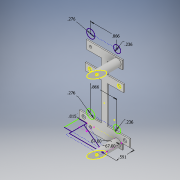
# Autodesk Inventor part: PI Rfid baracke angled reconfig
Saved by Autodesk Inventor 2018 (Build 220112000, 112)
## iProperties
Created: 2019-09-27
Part Number: PI Rfid baracke angled reconfig
Material: Generic
Document SubType Name: Modeling
Designer: Jacob
Density: 1 g/cm^3
Appearance: Default
Author: Jacob
Autodesk Inventor part; units mm, degrees
ref_plane "YZ Plane" through (0, 0, 0) normal (1, 0, 0) x (0, 1, 0)
ref_plane "XZ Plane" through (0, 0, 0) normal (0, 1, 0) x (-1, 0, 0)
ref_plane "XY Plane" through (0, 0, 0) normal (0, 0, 1) x (1, 0, 0)
sketch "Sketch1" plane through (0, 0, 0) normal (0, 0, 1) x (1, 0, 0)
  line L0 (-2.5, 15.5) -> (2.5, 15.5)
  line L1 (2.5, 15.5) -> (2.5, -15.5)
  line L2 (2.5, -15.5) -> (-2.5, -15.5)
  line L3 (-2.5, -15.5) -> (-2.5, 15.5)
  line L4 (-2.5, 15.5) -> (2.5, -15.5) construction
  line L5 (2.5, 15.5) -> (-2.5, -15.5) construction
  line L6 (0, 0) -> (0, 29.5852) construction
  line L7 (-16, 21.5) -> (16, 21.5)
  line L8 (16, 21.5) -> (16, 15.5)
  line L9 (16, 15.5) -> (-16, 15.5)
  line L10 (-16, 15.5) -> (-16, 21.5)
  line L11 (-16, 21.5) -> (16, 15.5) construction
  line L12 (16, 21.5) -> (-16, 15.5) construction
  line L13 (0, 0) -> (0, -27.9929) construction
  line L14 (-21, -15.5) -> (21, -15.5)
  line L15 (21, -15.5) -> (21, -21.5)
  line L16 (21, -21.5) -> (-21, -21.5)
  line L17 (-21, -21.5) -> (-21, -15.5)
  line L18 (-21, -15.5) -> (21, -21.5) construction
  line L19 (21, -15.5) -> (-21, -21.5) construction
  line L20 (16, 18.5) -> (-16, 18.5) construction
  line L21 (21, -18.5) -> (-21, -18.5) construction
  point P0 (0, 18.5)
  point P1 (0, -18.5)
  dimension "d0" = 5
  dimension "d2" = 32
  dimension "d3" = 6
  dimension "d4" = 0
  dimension "d5" = 42
  dimension "d6" = 6
  dimension "d7" = 0
  dimension "d65" = 37
  constraints: 44 end point, 10 midpoint, 7 parallel, 3 horizontal, 3 perpendicular, 2 point on line, 1 vertical
  measures "d0" distance between parallel lines of L1 L3
  measures "d2" distance of L7.start L7.end
  measures "d3" distance of L7.end L8.end
  measures "d4" distance between parallel lines of L0 L9
  measures "d5" distance of L15.end L16.end
  measures "d6" distance of L14.end L15.end
  measures "d7" distance between parallel lines of L2 L14
  measures "d65" vertical distance of L21.start L20.start
extrude "Extrusion1" add sketch "Sketch1" along normal blind 1
sketch "Sketch2" plane through (0, 0, 1) normal (0, 0, 1) x (1, 0, 0)
  line L0 (-16, 21.5) -> (-16, 15.5) projected
  line L1 (-16, 18.5) -> (16, 18.5) construction
  line L2 (16, 15.5) -> (16, 21.5) projected
  line L3 (-21, -15.5) -> (-21, -21.5) projected
  line L4 (-21, -18.5) -> (21, -18.5) construction
  line L5 (21, -15.5) -> (21, -21.5) projected
  circle A0 centre (-17.25, -18.5) radius 1.5
  circle A1 centre (17.25, -18.5) radius 1.5
  line L6 (0, 0) -> (0, -21.5) construction
  line L7 (21, -21.5) -> (-21, -21.5) projected
  line L8 (0, 0) -> (0, 21.5) construction
  line L9 (16, 21.5) -> (-16, 21.5) projected
  circle A2 centre (-12.25, 18.5) radius 1.5
  circle A3 centre (12.25, 18.5) radius 1.5
  dimension "d10" = 34.5
  dimension "d13" = 17.25
  dimension "d14" = 17.25
  dimension "d15" = 3
  dimension "d16" = 3
  dimension "d17" = 24.5
  dimension "d18" = 12.25
  dimension "d19" = 12.25
  dimension "d20" = 3
  dimension "d21" = 3
  dimension "d66" = 37
  constraints: 8 end point, 6 midpoint, 4 centre point, 4 point on line
  measures "d10" distance of A1.centre A0.centre
  measures "d13" distance from line of L6 A0.centre
  measures "d14" distance from line of L6 A1.centre
  measures "d15" diameter of A0
  measures "d16" diameter of A1
  measures "d17" distance of A3.centre A2.centre
  measures "d18" distance from line of L8 A2.centre
  measures "d19" distance from line of L8 A3.centre
  measures "d20" diameter of A2
  measures "d21" diameter of A3
  measures "d66" distance between parallel lines of L4 L1
extrude "Extrusion2" cut sketch "Sketch2" against normal blind 2
sketch "Sketch4" plane through (0, 0, 1) normal (0, 0, 1) x (1, 0, 0)
  line L0 (0, 0) -> (0, 68.1033) construction
  line L1 (0, 0) -> (0, -40.1743) construction
  line L2 (-15, 38.5) -> (15, 38.5)
  line L3 (15, 38.5) -> (15, 31.5)
  line L4 (15, 31.5) -> (-15, 31.5)
  line L5 (-15, 31.5) -> (-15, 38.5)
  line L6 (-15, 38.5) -> (15, 31.5) construction
  line L7 (15, 38.5) -> (-15, 31.5) construction
  line L8 (-15, -19.5) -> (15, -19.5)
  line L9 (15, -19.5) -> (15, -26.5)
  line L10 (15, -26.5) -> (-15, -26.5)
  line L11 (-15, -26.5) -> (-15, -19.5)
  line L12 (-15, -19.5) -> (15, -26.5) construction
  line L13 (15, -19.5) -> (-15, -26.5) construction
  circle A0 centre (-17.25, -18.5) radius 1.5 projected
  line L14 (-2.5, 31.5) -> (2.5, 31.5)
  line L15 (2.5, 31.5) -> (2.5, 21.5)
  line L16 (2.5, 21.5) -> (-2.5, 21.5)
  line L17 (-2.5, 21.5) -> (-2.5, 31.5)
  line L18 (-2.5, 31.5) -> (2.5, 21.5) construction
  line L19 (2.5, 31.5) -> (-2.5, 21.5) construction
  line L20 (16, 21.5) -> (-16, 21.5) projected
  line L21 (-15, -23) -> (15, -23) construction
  line L22 (-15, 35) -> (15, 35) construction
  circle A1 centre (-11.5, -23) radius 1
  circle A2 centre (11.5, -23) radius 1
  circle A3 centre (-11.5, 35) radius 1
  circle A4 centre (11.5, 35) radius 1
  line L23 (-16, 15.5) -> (-2.5, 15.5) projected
  point P0 (0, 35)
  point P1 (0, -23)
  point P2 (0, 26.5)
  dimension "d28" = 58
  dimension "d30" = 0
  dimension "d31" = 0
  dimension "d32" = 5
  dimension "d33" = 30
  dimension "d34" = 30
  dimension "d35" = 7
  dimension "d36" = 7
  dimension "d37" = 2
  dimension "d38" = 2
  dimension "d39" = 2
  dimension "d40" = 2
  dimension "d41" = 23
  dimension "d42" = 23
  dimension "d43" = 11.5
  dimension "d44" = 11.5
  dimension "d45" = 11.5
  dimension "d46" = 11.5
  dimension "d116" = 35
  constraints: 44 end point, 10 midpoint, 7 point on line, 6 parallel, 4 centre point, 3 horizontal, 3 perpendicular, 2 vertical
  measures "d28" distance of point (0, -23) point (0, 35)
  measures "d30" distance between parallel lines of L20 L16
  measures "d31" distance between parallel lines of L4 L14
  measures "d32" distance between parallel lines of L15 L17
  measures "d33" distance between parallel lines of L9 L11
  measures "d34" distance between parallel lines of L3 L5
  measures "d35" distance of L2.end L3.end
  measures "d36" distance of L8.end L9.end
  measures "d37" diameter of A3
  measures "d38" diameter of A4
  measures "d39" diameter of A1
  measures "d40" diameter of A2
  measures "d41" distance of A2.centre A1.centre
  measures "d42" distance of A4.centre A3.centre
  measures "d43" distance from line of L0 A3.centre
  measures "d44" distance from line of L0 A4.centre
  measures "d45" distance from line of L1 A1.centre
  measures "d46" distance from line of L1 A2.centre
  measures "d116" distance between parallel lines of L23 L8
extrude "Extrusion3" add sketch "Sketch4" against normal blind 1 contours L2 L3 L4 L5 | L4 L15 L16 L17 | L8 L9 L10 L11
sketch "Sketch5" plane through (0, 0, 1) normal (0, 0, 1) x (1, 0, 0)
  circle A0 centre (-12.25, 18.5) radius 1.5 projected
  circle A1 centre (12.25, 18.5) radius 1.5 projected
  circle A2 centre (-11.5, -13.5) radius 3.5
  circle A3 centre (-11.5, 44.5) radius 3.5
  line L0 (-11.5, -13.5) -> (11.5, -13.5) construction
  circle A4 centre (10.5, -13.5) radius 3
  line L1 (-11.5, 44.5) -> (11.5, 44.5) construction
  circle A5 centre (10.5, 44.5) radius 3
  point P0 (0, 0)
  dimension "d52" = 7
  dimension "d55" = 7
  dimension "d97" = 6
  dimension "d98" = 22
  dimension "d99" = 6
  dimension "d100" = 22
  constraints: 4 centre point, 4 end point, 2 horizontal, 2 point on line, 1 coincident
  measures "d52" diameter of A2
  measures "d55" diameter of A3
  measures "d97" diameter of A4
  measures "d98" distance of A4.centre A2.centre
  measures "d99" diameter of A5
  measures "d100" distance of A5.centre A3.centre
extrude "Extrusion5" [suppressed]
sketch "Sketch6" plane through (0, 0, 0) normal (0, 0, -1) x (-1, 0, 0)
  circle A0 centre (-17.25, -18.5) radius 1.5 projected
  circle A1 centre (-17.25, -18.5) radius 3
  circle A2 centre (17.25, -18.5) radius 1.5 projected
  circle A3 centre (17.25, -18.5) radius 3
  circle A4 centre (12.25, 18.5) radius 1.5 projected
  circle A5 centre (12.25, 18.5) radius 3
  circle A6 centre (-12.25, 18.5) radius 1.5 projected
  circle A7 centre (-12.25, 18.5) radius 3
  point P0 (0, 0)
  dimension "d59" = 6
  dimension "d60" = 6
  dimension "d61" = 6
  dimension "d62" = 6
  constraints: 4 centre point, 4 coincident
  measures "d59" diameter of A7
  measures "d60" diameter of A5
  measures "d61" diameter of A1
  measures "d62" diameter of A3
extrude "Extrusion6" [suppressed]
sketch "Sketch8" plane through (-21, -21.5, 0) normal (0, -1, 0) x (1, 0, 0)
  line L0 (35.5, 13.7) -> (29.5, 13.7) construction
  line L1 (35.5, 1) -> (35.5, 13.7) construction
  line L2 (29.5, 1) -> (29.5, 13.7) construction
  line L3 (6.5, 1) -> (6.5, 7.35) construction
  line L4 (12.5, 7.35) -> (6.5, 7.35) construction
  line L5 (12.5, 1) -> (12.5, 7.35) construction
  line L6 (0, 1) -> (42, 1) construction
  line L7 (35.5, 13.7) -> (6.5, 1.3902) construction
  line L8 (35.5, 13.7) -> (6.5, 13.7) construction
  line L9 (6.5, 13.7) -> (6.5, 1.3902) construction
  line L10 (6.5, 13.7) -> (0, 13.7)
  line L11 (0, 13.7) -> (0, 1.3902)
  line L12 (0, 1.3902) -> (6.5, 1.3902)
  line L13 (6.5, 1.3902) -> (6.5, 13.7)
  line L14 (35.5, 13.7) -> (35.5, 18.3) construction
  line L15 (6.5, 13.7) -> (6.5, 18.3) construction
  line L16 (6.5, 18.3) -> (35.5, 18.3) construction
  line L17 (35.5, 16) -> (6.5, 16)
  line L18 (35.5, 16) -> (6.5, 3.6902)
  line L19 (6.5, 16) -> (6.5, 3.6902)
  point P0 (21, 0)
  dimension "d72" = 67
  dimension "d139" = 0.3902
  dimension "d140" = 15
  dimension "d141" = 67
  constraints: 26 end point, 3 vertical, 2 horizontal, 2 midpoint, 2 parallel, 2 perpendicular, 2 point on line, 1 collinear
  measures "d72" angle of L1 L7
  measures "d139" distance between parallel lines of L6 L12
  measures "d140" distance between parallel lines of L6 L17
  measures "d141" angle of L14 L18
extrude "Extrusion9" [suppressed]
extrude "Extrusion14" [suppressed]
sketch "Sketch13" plane through (0, 0, 1) normal (0, 0, 1) x (1, 0, 0)
  circle A0 centre (-11.5, -23) radius 1 projected
  circle A1 centre (11.5, -23) radius 1 projected
  line L0 (-11.5, -23) -> (11.5, -23) construction
  circle A2 centre (-11.5, 35) radius 1 projected
  circle A3 centre (11.5, 35) radius 1 projected
  line L1 (-11.5, 35) -> (11.5, 35) construction
  circle A4 centre (-11, 35) radius 3
  circle A5 centre (11, 35) radius 3
  circle A6 centre (-11, -23) radius 3
  circle A7 centre (11, -23) radius 3
  line L2 (0, 35) -> (0, -23) construction
  point P0 (0, 0)
  dimension "d43" = 11.5
  dimension "d44" = 11.5
  dimension "d45" = 11.5
  dimension "d46" = 11.5
  dimension "d117" = 6
  dimension "d118" = 6
  dimension "d119" = 6
  dimension "d120" = 6
  dimension "d121" = 22
  dimension "d122" = 22
  dimension "d123" = 11
  dimension "d124" = 11
  dimension "d125" = 11
  dimension "d126" = 11
  constraints: 6 end point, 4 centre point, 4 point on line, 2 horizontal, 2 midpoint
  measures "d117" diameter of A4
  measures "d118" diameter of A5
  measures "d119" diameter of A6
  measures "d120" diameter of A7
  measures "d121" distance of A7.centre A6.centre
  measures "d122" distance of A5.centre A4.centre
  measures "d123" distance of L2.start A4.centre
  measures "d124" distance of L2.start A5.centre
  measures "d125" distance of L2.end A6.centre
  measures "d126" distance of L2.end A7.centre
extrude "Extrusion19" add sketch "Sketch13" along normal blind 22.86 contours A1 | A3 | A5 | A7
sketch "Sketch16" plane through (-15, -26.5, 1) normal (0, -1, 0) x (1, 0, 0)
  line L0 (29, 22.86) -> (23, 22.86) projected
  line L1 (23, 22.86) -> (35.7, 22.86)
  line L2 (36, 0) -> (17.5, 0) projected
  line L3 (36, 0) -> (35.7, 0)
  line L4 (35.7, 0) -> (35.7, 22.86)
  line L5 (23, 22.86) -> (35.7, 0)
  point P0 (15, -1)
  dimension "d155" = 12.7
  dimension "d163" = 60.945
  constraints: 8 end point, 2 horizontal, 1 perpendicular
  measures "d155" distance of L0.end L1.end
  measures "d163" angle of L5 L1
extrude "Extrusion20" cut sketch "Sketch16" against normal blind 127
sketch "Sketch17" plane through (11, -23, 18.46) normal (0.8741573, 0, 0.4856429) x (0.4856429, 0, -0.8741573)
  ellipse E0 centre (0, 0) end of major axis (-6.1774, 0) minor radius 3 projected
  ellipse E1 centre (0, 58) end of major axis (-6.1774, 58) minor radius 3 projected
  line L0 (0, -3) -> (0, 61) construction
  circle A0 centre (0, 0) radius 1
  ellipse E2 centre (4.3358, 58) end of major axis (4.3358, 59) minor radius 0.4856 projected
  circle A1 centre (0, 58) radius 1
  point P0 (10.7949, 23)
  dimension "d160" = 2
  dimension "d162" = 2
  constraints: 2 centre point, 2 coincident, 2 end point, 2 vertical alignment, 1 vertical, 3 other
  measures "d160" diameter of A0
  measures "d162" diameter of A1
extrude "Extrusion21" cut sketch "Sketch17" against normal blind 5 contours A0 | A1
sketch "Sketch18" plane through (11, -23, 18.46) normal (0.8741573, 0, 0.4856429) x (0.4856429, 0, -0.8741573)
  ellipse E0 centre (0, 0) end of major axis (-6.1774, 0) minor radius 3 projected
  circle A0 centre (0, 0) radius 1 projected
  ellipse E1 centre (0, 58) end of major axis (-6.1774, 58) minor radius 3 projected
  circle A1 centre (0, 58) radius 1 projected
  point P0 (10.7949, 23)
  constraints: 2 other
equation "\"d13\" = d14"
equation "\"d18\" = d19"
equation "\"d43\" = d44"
equation "\"d45\" = d46"
equation "\"d123\" = d124"
equation "\"d125\" = d126"
body "Solid1"
